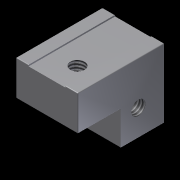
# Autodesk Inventor part: 3. Leiterplattenhalter_Rechts
Saved by Autodesk Inventor 2011 SP1 (Build 150282100, 282)
## iProperties
Created: 2012-05-07
Part Number: 3. Leiterplattenhalter_Rechts
Document SubType Name: Modeling
Designer: pburkhar
Density: 1 g/cm^3
Author: pburkhar
Autodesk Inventor part; units mm, degrees
ref_plane "YZ Plane" through (0, 0, 0) normal (1, 0, 0) x (0, 1, 0)
ref_plane "XZ Plane" through (0, 0, 0) normal (0, 1, 0) x (-1, 0, 0)
ref_plane "XY Plane" through (0, 0, 0) normal (0, 0, 1) x (1, 0, 0)
sketch "Skizze1" plane through (0, 0, 0) normal (0, 0, 1) x (1, 0, 0)
  line L0 (0, 12.3) -> (8.8, 12.3)
  line L1 (0, 12.3) -> (0, 0)
  line L2 (0, 0) -> (8.8, 0)
  line L3 (8.8, 0) -> (8.8, 12.3)
  circle A0 centre (5.18, 3.55) radius 1.25
  circle A1 centre (5.18, 3.55) radius 1.25
  line L4 (0, 12.3) -> (8.8, 12.3)
  line L5 (8.8, 12.3) -> (8.8, 0)
  line L6 (8.8, 0) -> (0, 0)
  line L7 (0, 0) -> (0, 12.3)
  dimension "d35" = 8.8
  dimension "d36" = 5.18
  constraints: 16 end point, 2 centre point, 2 parallel, 1 coincident, 1 concentric, 1 horizontal, 1 perpendicular
  measures "d35" distance between parallel lines of L1 L3
  measures "d36" distance from line of L1 A0.centre
extrude "Extrusion1" add sketch "Skizze1" along normal blind 9.8
sketch "Skizze2" plane through (8.8, 0, 0) normal (1, 0, 0) x (0, 0, -1)
  line L0 (0, 0) -> (-9.8, 0) projected
  line L1 (0, 0) -> (0, 12.3) projected
  line L2 (0, 12.3) -> (-9.8, 12.3) projected
  line L3 (-4.8, 6.1) -> (0, 6.1)
  line L4 (0, 6.1) -> (0, 0)
  line L5 (0, 0) -> (-4.8, 0)
  line L6 (-4.8, 0) -> (-4.8, 6.1)
  dimension "d2" = 6.2
  dimension "d3" = 4.8
  dimension "d4" = 6.1
  constraints: 8 end point, 2 parallel, 1 horizontal, 1 perpendicular
  measures "d2" distance between parallel lines of L2 L3
  measures "d3" distance between parallel lines of L1 L6
  measures "d4" distance between parallel lines of L3 L0
extrude "Extrusion2" cut sketch "Skizze2" against normal blind 9.8
sketch "Skizze3" plane through (8.8, 0, 9.8) normal (1, 0, 0) x (0, 0, -1)
  line L0 (9.8, 6.1) -> (9.8, 12.3) projected
  line L1 (9.8, 12.3) -> (0, 12.3) projected
  point P0 (9.8, 0)
  point P1 (6.1, 8.6)
  dimension "d7" = 3.7
  dimension "d8" = 3.7
  measures "d7" distance from line of L1 point (6.1, 8.6)
  measures "d8" distance from line of L0 point (6.1, 8.6)
hole "Hole1" at (8.8, 8.6, 3.7) direction (-1, 0, 0) diameter 2.013 end through all thread size "M2.5x0.45" class "6H" standard "ANSI Metric M Profile"
sketch "Skizze4" plane through (0, 0, 9.8) normal (0, 0, 1) x (1, 0, 0)
  circle A0 centre (5.18, 3.55) radius 1.25 projected
  circle A1 centre (5.18, 3.55) radius 1.25
  constraints: 1 centre point, 1 coincident, 1 concentric
extrude "Extrusion3" add sketch "Skizze4" against normal blind 5
sketch "Skizze5" plane through (0, 0, 9.8) normal (0, 0, 1) x (1, 0, 0)
  line L0 (8.8, 0) -> (0, 0) projected
  line L1 (8.8, 12.3) -> (8.8, 0) projected
  point P0 (5.2, 3.55)
  dimension "d18" = 3.6
  dimension "d19" = 3.55
  measures "d18" distance from line of L1 point (5.2, 3.55)
  measures "d19" distance from line of L0 point (5.2, 3.55)
hole "Hole2" at (5.2, 3.55, 9.8) direction (0, 0, -1) diameter 2.013 depth 8 tip angle 118 thread size "M2.5x0.45" class "6H" standard "ANSI Metric M Profile"
fillet "Rundung1" radius 0.2 1 edges at (0, 12.3, 4.9)
fillet "Rundung2" radius 0.1 18 edges at (0, 9.1, 0) (0.0586, 12.2414, 0) (4.5, 12.3, 0) (0, 6.1, 2.4) (0, 3.05, 4.8) (4.4, 0, 4.8) (4.4, 6.1, 4.8) (4.4, 6.1, 0) (8.8, 9.2, 0) (8.8, 3.05, 4.8) (8.8, 0, 7.3) (0, 0, 7.3) (8.8, 12.3, 4.9) (8.8, 6.15, 9.8) (4.4, 0, 9.8) (0, 6.05, 9.8) (0.0586, 12.2414, 9.8) (4.5, 12.3, 9.8)
sketch "Skizze6" plane through (0.1, 0, 9.7) normal (0, -1, 0) x (1, 0, 0)
  line L0 (8.6, 0.1) -> (0, 0.1) projected
  line L1 (-0.1, 0) -> (-0.1, -4.8) projected
  line L2 (8.7, -4.8) -> (8.7, 0) projected
  line L3 (1.699, 0.1) -> (6.901, 0.1)
  line L4 (6.901, 0.1) -> (6.901, -0.1)
  line L5 (6.901, -0.1) -> (1.699, -0.1)
  line L6 (1.699, -0.1) -> (1.699, 0.1)
  point P0 (-0.1, -9.7)
  dimension "d30" = 0.2
  dimension "d31" = 1.799
  dimension "d32" = 1.799
  constraints: 8 end point, 2 parallel, 1 horizontal, 1 perpendicular, 1 point on line
  measures "d30" distance between parallel lines of L5 L3
  measures "d31" distance from line of L1 L5.end
  measures "d32" horizontal distance of L2.end L3.end
extrude "Extrusion4" cut sketch "Skizze6" against normal blind 12.5
